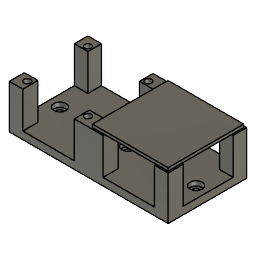
H bridge Mount Front (Autodesk Fusion 360 design; units mm, degrees)
Autodesk Fusion 360 part; units mm, degrees
note: some values were not read from the file. Set by a fixed rule: which face or edge a step refers to.
sketch "Skizze2" plane through (0, 0, 0) normal (0, 0, 1) x (1, 0, 0)
  line L0 (1.5, -1) -> (51.5, -1) construction
  line L1 (51.5, -1) -> (51.5, -51) construction
  line L2 (51.5, -51) -> (1.5, -51) construction
  line L3 (1.5, -51) -> (1.5, -1) construction
  line L4 (-1.5, -1) -> (-51.5, -1) construction
  line L5 (-51.5, -1) -> (-51.5, -51) construction
  line L6 (-51.5, -51) -> (-1.5, -51) construction
  line L7 (-1.5, -51) -> (-1.5, -1) construction
  line L8 (1.5, -1) -> (-1.5, -1) construction
  line L9 (1.5, -1) -> (51.5, -51) construction
  line L10 (-1.5, -1) -> (-51.5, -51) construction
  line L11 (46.5, -6) -> (6.5, -6) construction
  line L12 (6.5, -6) -> (6.5, -46) construction
  line L13 (6.5, -46) -> (46.5, -46) construction
  line L14 (46.5, -46) -> (46.5, -6) construction
  line L15 (46.5, -6) -> (6.5, -46) construction
  line L16 (6.5, -6) -> (46.5, -46) construction
  line L17 (52.5, 0) -> (-52.5, 0)
  line L18 (-52.5, 0) -> (-52.5, -52)
  line L19 (-52.5, -52) -> (52.5, -52)
  line L20 (52.5, -52) -> (52.5, 0)
  line L21 (52.5, 0) -> (43.5, 0)
  line L22 (43.5, 0) -> (43.5, -9)
  line L23 (43.5, -9) -> (52.5, -9)
  line L24 (52.5, -9) -> (52.5, 0)
  circle A0 centre (46.5, -6) radius 2.15
  line L25 (26.5, -26) -> (26.5, 0) construction
  circle A1 centre (6.5, -6) radius 2.15
  line L26 (9.5, -9) -> (0.5, -9)
  line L27 (9.5, 0) -> (9.5, -9)
  line L28 (0.5, -9) -> (0.5, 0)
  line L29 (0.5, 0) -> (9.5, 0)
  line L30 (26.5, -26) -> (11, -26) construction
  circle A2 centre (46.5, -46) radius 2.15
  line L31 (43.5, -43) -> (52.5, -43)
  line L32 (43.5, -52) -> (43.5, -43)
  line L33 (9.5, -43) -> (0.5, -43)
  line L34 (9.5, -52) -> (9.5, -43)
  circle A3 centre (6.5, -46) radius 2.15
  line L35 (0.5, -43) -> (0.5, -52)
  line L36 (0, 0) -> (0, -52)
  point P0 (0, -1)
  point P1 (26.5, -26)
  dimension "d2" = 50
  dimension "d3" = 50
  dimension "d4" = 3
  dimension "d5" = 40
  dimension "d6" = 1
  dimension "d7" = 1
  dimension "d8" = 1
  dimension "d9" = 1
  dimension "d10" = 8
  dimension "d11" = 4.3
  constraint horizontal L0
  constraint vertical L1
  constraint horizontal L2
  constraint vertical L3
  constraint horizontal L4
  constraint vertical L5
  constraint horizontal L6
  constraint vertical L7
  constraint horizontal L2.end L6.end
  constraint horizontal L0.start L4.start
  constraint equal L6 L7
  constraint midpoint L8 P0
  constraint vertical L36.start P0
  constraint horizontal L11
  constraint perpendicular L11 L12
  constraint parallel L11 L13
  constraint parallel L12 L14
  constraint coincident L15 P1
  constraint coincident L16 P1
  constraint midpoint L9 P1
  constraint equal L13 L14
  constraint horizontal L17
  constraint vertical L18
  constraint horizontal L19
  constraint vertical L20
  constraint horizontal L21
  constraint vertical L22
  constraint horizontal L23
  constraint vertical L24
  constraint coincident L15 L22.end
  constraint coincident L11.start L14.end
  constraint coincident P1 L25.start
  constraint coincident L17 L25.end
  constraint perpendicular L17 L25
  constraint symmetric L17.start L25 L28.end
  constraint symmetric L21.end L25 L27.start
  constraint symmetric L22.end L25 L26.start
  constraint symmetric L23.end L25 L26.end
  constraint symmetric A0 L25 A1
  constraint coincident L36.start L17
  constraint horizontal L30
  constraint symmetric L21.end L30 L32.start
  constraint symmetric L22.end L30 L31.start
  constraint symmetric L23.end L30 L31.end
  constraint symmetric A0 L30 A2
  constraint symmetric A1 L30 A3
  constraint symmetric L26.start L30 L33.start
  constraint symmetric L26.end L30 L33.end
  constraint symmetric L27.start L30 L34.start
  constraint coincident L19 L35.end
  constraint perpendicular L19 L35
  constraint coincident L36.start origin
  constraint midpoint L19 L36.end
  measures "d2" distance of L0.start L0.end
  measures "d3" distance of L0.start L2.end
  measures "d4" distance of L0.start L4.start
  measures "d5" distance of L11.end L12.end
  measures "d6" distance of L36.start P0
  measures "d7" distance of L2 L19
  measures "d8" distance of L1 L20
  measures "d9" distance of L5 L18
  measures "d10" distance of L0 L23
  measures "d11" diameter of A0
extrude "Extrusion1" add sketch "Skizze2" against normal blind 5 contours L17 L20 L21 L22 L23 L24 | L17 L19 L20 L22 L23 L26 L27 L28 L31 L32 L33 L34 L35 L36 | L17 L26 L27 L28 L29 | L19 L20 L31 L32 | L19 L33 L34 L35 | A0 | A1 | A2 | A3 makes body 1
extrude "Extrusion2" add sketch "Skizze2" along normal blind 24 contours L17 L20 L21 L22 L23 L24 | L17 L26 L27 L28 L29 | L19 L20 L31 L32 | L19 L33 L34 L35 bodies 1
extrude "Extrusion3" add sketch "Skizze2" along normal up to surface (14 mm away) contours A0 | A1 | A2 | A3 bodies 1
sketch "Skizze4" plane through (0, 0, 24) normal (0, 0, 1) x (-1, 0, 0)
  circle A0 centre (-46.5, 46) radius 2.15
  line L0 (-52.5, 52) -> (-52.5, 43)
  line L1 (-52.5, 43) -> (-43.5, 43)
  line L2 (-43.5, 43) -> (-43.5, 52)
  line L3 (-43.5, 52) -> (-52.5, 52)
  circle A1 centre (-6.5, 46) radius 2.15 construction
  circle A2 centre (-46.5, 6) radius 2.15 construction
  line L4 (-6.5, 46) -> (-46.5, 6) construction
  line L5 (-1.5, 51) -> (-51.5, 51)
  line L6 (-51.5, 51) -> (-51.5, 1)
  line L7 (-51.5, 1) -> (-1.5, 1)
  line L8 (-1.5, 1) -> (-1.5, 51)
  line L9 (-1.5, 51) -> (-51.5, 1) construction
  line L10 (-51.5, 51) -> (-1.5, 1) construction
  point P0 (-9.5, 43)
  point P1 (-43.5, 9)
  point P2 (-26.5, 26)
  dimension "d29" = 50
  dimension "d30" = 50
  constraint coincident A1.centre L4.start
  constraint coincident A2.centre L4.end
  constraint horizontal L5
  constraint perpendicular L5 L6
  constraint parallel L5 L7
  constraint parallel L6 L8
  constraint coincident L9 P2
  constraint coincident L10 P2
  constraint midpoint L4 P2
  measures "d29" distance of L6.end L7.end
  measures "d30" distance of L5.end L6.end
extrude "Extrusion5" add sketch "Skizze4" along normal blind 2 separate body contours A0 | L1 L2 L5 L6 | L1 L2 L5 L6 L7 L8 makes body 2
mirror "Spiegeln1" about plane through (0, 0, 0) normal (-1, 0, 0) of bodies 1 merged
extrude "Extrusion19" add 4 faces at (6.5, -43, 8) (-6.5, -43, 8) (-49.5, -43, 16) (49.5, -43, 16) along direction (0, 1, 0) blind 1 on bodies 1 bodies 1
sketch "Skizze12" plane through (0, 0, 0) normal (0, 0, 1) x (-1, 0, 0)
  line L0 (-9.5, 42) -> (-9.5, 52)
  line L1 (0.5, 52) -> (-0.5, 52)
  line L2 (-43.5, 52) -> (-43.5, 42)
  line L3 (-52.5, 42) -> (-52.5, 9)
  line L4 (-52.5, 9) -> (-43.5, 9)
  line L5 (-43.5, 9) -> (-43.5, 0)
  line L6 (-43.5, 0) -> (-9.5, 0)
  line L7 (-9.5, 0) -> (-9.5, 9)
  line L8 (-9.5, 9) -> (-0.5, 9)
  line L9 (9.5, 9) -> (9.5, 0)
  line L10 (43.5, 0) -> (43.5, 9)
  line L11 (43.5, 9) -> (52.5, 9)
  line L12 (52.5, 9) -> (52.5, 42)
  line L13 (43.5, 42) -> (43.5, 52)
  line L14 (43.5, 52) -> (9.5, 52)
  line L15 (9.5, 52) -> (9.5, 42)
  line L16 (-43.5, 42) -> (-52.5, 42)
  circle A0 centre (-45, 26) radius 2.1
  circle A1 centre (0, 26) radius 2.1
  circle A2 centre (45, 26) radius 2.1
  line L17 (-45, 26) -> (45, 26) construction
  circle A3 centre (-45, 26) radius 4
  circle A4 centre (0, 26) radius 4
  circle A5 centre (45, 26) radius 4
  line L18 (0, 0) -> (0, 52) construction
  line L19 (9.5, 0) -> (43.5, 0)
  line L20 (52.5, 42) -> (43.5, 42)
  line L21 (-0.5, 9) -> (-0.5, 0)
  line L22 (-0.5, 0) -> (0.5, 0)
  line L23 (0.5, 0) -> (0.5, 9)
  line L24 (0.5, 9) -> (9.5, 9)
  line L25 (9.5, 42) -> (0.5, 42)
  line L26 (0.5, 42) -> (0.5, 52)
  line L27 (-0.5, 52) -> (-0.5, 42)
  line L28 (-0.5, 42) -> (-9.5, 42)
  line L29 (-9.5, 52) -> (-43.5, 52)
  dimension "d84" = 90
  dimension "d85" = 4.2
  dimension "d86" = 8
  constraint coincident A0.centre L17.start
  constraint coincident A2.centre L17.end
  constraint horizontal L17
  constraint midpoint A1.centre L17
  constraint vertical L18.start A1.centre
  constraint concentric A0 A3
  constraint concentric A1 A4
  constraint concentric A2 A5
  constraint equal A0 A1
  constraint equal A0 A2
  constraint equal A4 A5
  constraint equal A3 A4
  constraint coincident L18.start origin
  constraint parallel L12 L18
  constraint coincident L1 L18.end
  constraint midpoint A1.centre L18
  measures "d84" distance of A0.centre A2.centre
  measures "d85" diameter of A0
  measures "d86" diameter of A3
extrude "Extrusion20" cut sketch "Skizze12" against normal blind 3 contours A3 | A4 | A5 bodies 1
extrude "Extrusion21" cut 3 faces at (44.5562, -26.1724, 0) (0.6307, -25.6963, 0) (-45.4438, -26.1724, 0) along direction (0, 0, -1) through all on bodies 1 bodies 1
extrude "Extrusion23" add 2 faces at (-0.5, -45.3333, 8) (-0.5, -6, 8) along direction (1, 0, 0) up to surface end surface through (0.5, -43, 0) normal (-1, 0, 0) offset 0 on bodies 1 bodies 1
equation "d7 = d6"
equation "d8 = d6"
equation "d9 = d6"
